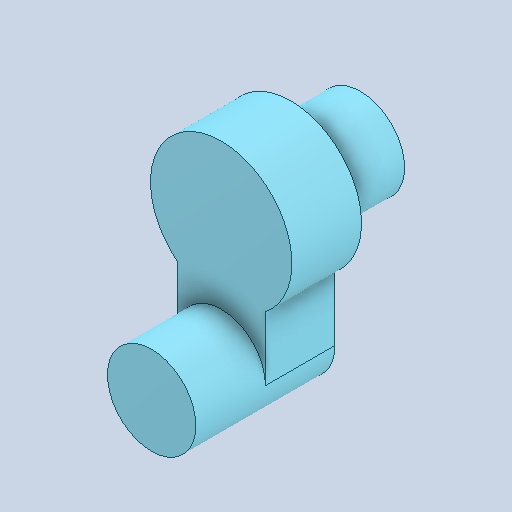
# Autodesk Inventor part: Component37
Saved by Autodesk Inventor 2022 (Build 260153000, 153)
## iProperties
Created: 2022-01-29
Part Number: Component37
Material: Generic
Document SubType Name: Modeling
Designer: Administrator
Density: 1 g/cm^3
Appearance: Default
Title: Component37
Author: Administrator
Autodesk Inventor part; units mm, degrees
ref_plane "YZ Plane" through (0, 0, 0) normal (1, 0, 0) x (0, 1, 0)
ref_plane "XZ Plane" through (0, 0, 0) normal (0, 1, 0) x (-1, 0, 0)
ref_plane "XY Plane" through (0, 0, 0) normal (0, 0, 1) x (1, 0, 0)
sketch "Sketch2" plane through (0, 0, 0) normal (0, 0, 1) x (1, 0, 0)
  arc A0 (3.175, -8.5584) -> (-3.175, -8.5584) centre (0, -8.5584) ccw
  line L0 (3.175, -3.9656) -> (3.175, -8.5584)
  arc A1 (3.175, -3.9656) -> (-3.175, -3.9656) centre (0, 0) ccw
  line L1 (-3.175, -8.5584) -> (-3.175, -3.9656)
  circle A2 centre (0, -8.5584) radius 3.175
  circle A3 centre (0, 0) radius 3.175
  point P0 (0, 0)
  point P1 (-3.175, -8.5584)
  point P2 (3.175, -8.5584)
  point P3 (-3.175, -8.5584)
  point P4 (3.175, -8.5584)
  constraints: 4 centre point, 4 end point, 4 point on circle
extrude "Extrusion1" add sketch "Sketch2" against normal blind 5 contours A2 A0 | A0 L1 A1 L0 | A3
extrude "Extrusion2" add sketch "Sketch2" along normal blind 5 contours A2 A0
sketch "Sketch3" plane through (0, 0, -5) normal (0, 0, -1) x (-1, 0, 0)
  circle A0 centre (0, 0) radius 3.175 projected
  point P0 (0, 0)
extrude "Extrusion3" add sketch "Sketch3" along normal blind 5
body "Solid1"
